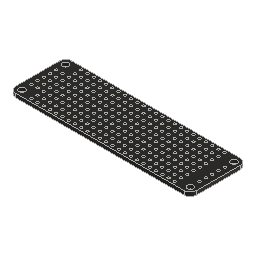
Ingenuity_Micro_Feather_Stacker (Autodesk Fusion 360 design; units mm, degrees)
Autodesk Fusion 360 part; units mm, degrees
sketch "Sketch1" plane through (0, 0, 0) normal (0, 0, 1) x (1, 0, 0) in component "Ingenuity_Micro_Feather_Wing"
  line L0 (36.83, 11.43) -> (-36.83, 11.43)
  line L1 (-36.83, 11.43) -> (-36.83, -11.43)
  line L2 (-36.83, -11.43) -> (36.83, -11.43)
  line L3 (36.83, -11.43) -> (36.83, 11.43)
  line L4 (36.83, 11.43) -> (-36.83, -11.43) construction
  line L5 (-36.83, 11.43) -> (36.83, -11.43) construction
  circle A0 centre (-34.29, 8.89) radius 1.27
  circle A1 centre (-34.29, -8.89) radius 1.27
  line L6 (-36.83, 0) -> (36.83, 0) construction
  line L7 (0, 11.43) -> (0, -11.43) construction
  circle A2 centre (34.29, 8.89) radius 1.27
  circle A3 centre (34.29, -8.89) radius 1.27
  circle A4 centre (-34.29, 0) radius 0.51
  line L8 (-34.29, 8.89) -> (-34.29, -8.89) construction
  circle A5 centre (-34.29, -5.08) radius 0.51
  circle A6 centre (-31.75, -5.08) radius 0.51
  circle A7 centre (-34.29, -2.54) radius 0.51
  circle A8 centre (-31.75, -2.54) radius 0.51
  circle A9 centre (-31.75, 0) radius 0.51
  circle A10 centre (-34.29, 2.54) radius 0.51
  circle A11 centre (-31.75, 2.54) radius 0.51
  circle A12 centre (-34.29, 5.08) radius 0.51
  circle A13 centre (-31.75, 5.08) radius 0.51
  circle A14 centre (-29.21, 0) radius 0.51
  circle A15 centre (-29.21, -10.16) radius 0.51
  circle A16 centre (-26.67, -10.16) radius 0.51
  circle A17 centre (-24.13, -10.16) radius 0.51
  circle A18 centre (-21.59, -10.16) radius 0.51
  circle A19 centre (-19.05, -10.16) radius 0.51
  circle A20 centre (-16.51, -10.16) radius 0.51
  circle A21 centre (-13.97, -10.16) radius 0.51
  circle A22 centre (-11.43, -10.16) radius 0.51
  circle A23 centre (-8.89, -10.16) radius 0.51
  circle A24 centre (-6.35, -10.16) radius 0.51
  circle A25 centre (-3.81, -10.16) radius 0.51
  circle A26 centre (-1.27, -10.16) radius 0.51
  circle A27 centre (1.27, -10.16) radius 0.51
  circle A28 centre (3.81, -10.16) radius 0.51
  circle A29 centre (6.35, -10.16) radius 0.51
  circle A30 centre (8.89, -10.16) radius 0.51
  circle A31 centre (11.43, -10.16) radius 0.51
  circle A32 centre (13.97, -10.16) radius 0.51
  circle A33 centre (16.51, -10.16) radius 0.51
  circle A34 centre (19.05, -10.16) radius 0.51
  circle A35 centre (21.59, -10.16) radius 0.51
  circle A36 centre (24.13, -10.16) radius 0.51
  circle A37 centre (26.67, -10.16) radius 0.51
  circle A38 centre (29.21, -10.16) radius 0.51
  circle A39 centre (-29.21, -7.62) radius 0.51
  circle A40 centre (-26.67, -7.62) radius 0.51
  circle A41 centre (-24.13, -7.62) radius 0.51
  circle A42 centre (-21.59, -7.62) radius 0.51
  circle A43 centre (-19.05, -7.62) radius 0.51
  circle A44 centre (-16.51, -7.62) radius 0.51
  circle A45 centre (-13.97, -7.62) radius 0.51
  circle A46 centre (-11.43, -7.62) radius 0.51
  circle A47 centre (-8.89, -7.62) radius 0.51
  circle A48 centre (-6.35, -7.62) radius 0.51
  circle A49 centre (-3.81, -7.62) radius 0.51
  circle A50 centre (-1.27, -7.62) radius 0.51
  circle A51 centre (1.27, -7.62) radius 0.51
  circle A52 centre (3.81, -7.62) radius 0.51
  circle A53 centre (6.35, -7.62) radius 0.51
  circle A54 centre (8.89, -7.62) radius 0.51
  circle A55 centre (11.43, -7.62) radius 0.51
  circle A56 centre (13.97, -7.62) radius 0.51
  circle A57 centre (16.51, -7.62) radius 0.51
  circle A58 centre (19.05, -7.62) radius 0.51
  circle A59 centre (21.59, -7.62) radius 0.51
  circle A60 centre (24.13, -7.62) radius 0.51
  circle A61 centre (26.67, -7.62) radius 0.51
  circle A62 centre (29.21, -7.62) radius 0.51
  circle A63 centre (-29.21, -5.08) radius 0.51
  circle A64 centre (-26.67, -5.08) radius 0.51
  circle A65 centre (-24.13, -5.08) radius 0.51
  circle A66 centre (-21.59, -5.08) radius 0.51
  circle A67 centre (-19.05, -5.08) radius 0.51
  circle A68 centre (-16.51, -5.08) radius 0.51
  circle A69 centre (-13.97, -5.08) radius 0.51
  circle A70 centre (-11.43, -5.08) radius 0.51
  circle A71 centre (-8.89, -5.08) radius 0.51
  circle A72 centre (-6.35, -5.08) radius 0.51
  circle A73 centre (-3.81, -5.08) radius 0.51
  circle A74 centre (-1.27, -5.08) radius 0.51
  circle A75 centre (1.27, -5.08) radius 0.51
  circle A76 centre (3.81, -5.08) radius 0.51
  circle A77 centre (6.35, -5.08) radius 0.51
  circle A78 centre (8.89, -5.08) radius 0.51
  circle A79 centre (11.43, -5.08) radius 0.51
  circle A80 centre (13.97, -5.08) radius 0.51
  circle A81 centre (16.51, -5.08) radius 0.51
  circle A82 centre (19.05, -5.08) radius 0.51
  circle A83 centre (21.59, -5.08) radius 0.51
  circle A84 centre (24.13, -5.08) radius 0.51
  circle A85 centre (26.67, -5.08) radius 0.51
  circle A86 centre (29.21, -5.08) radius 0.51
  circle A87 centre (-29.21, -2.54) radius 0.51
  circle A88 centre (-26.67, -2.54) radius 0.51
  circle A89 centre (-24.13, -2.54) radius 0.51
  circle A90 centre (-21.59, -2.54) radius 0.51
  circle A91 centre (-19.05, -2.54) radius 0.51
  circle A92 centre (-16.51, -2.54) radius 0.51
  circle A93 centre (-13.97, -2.54) radius 0.51
  circle A94 centre (-11.43, -2.54) radius 0.51
  circle A95 centre (-8.89, -2.54) radius 0.51
  circle A96 centre (-6.35, -2.54) radius 0.51
  circle A97 centre (-3.81, -2.54) radius 0.51
  circle A98 centre (-1.27, -2.54) radius 0.51
  circle A99 centre (1.27, -2.54) radius 0.51
  circle A100 centre (3.81, -2.54) radius 0.51
  circle A101 centre (6.35, -2.54) radius 0.51
  circle A102 centre (8.89, -2.54) radius 0.51
  circle A103 centre (11.43, -2.54) radius 0.51
  circle A104 centre (13.97, -2.54) radius 0.51
  circle A105 centre (16.51, -2.54) radius 0.51
  circle A106 centre (19.05, -2.54) radius 0.51
  circle A107 centre (21.59, -2.54) radius 0.51
  circle A108 centre (24.13, -2.54) radius 0.51
  circle A109 centre (26.67, -2.54) radius 0.51
  circle A110 centre (29.21, -2.54) radius 0.51
  circle A111 centre (-26.67, 0) radius 0.51
  circle A112 centre (-24.13, 0) radius 0.51
  circle A113 centre (-21.59, 0) radius 0.51
  circle A114 centre (-19.05, 0) radius 0.51
  circle A115 centre (-16.51, 0) radius 0.51
  circle A116 centre (-13.97, 0) radius 0.51
  circle A117 centre (-11.43, 0) radius 0.51
  circle A118 centre (-8.89, 0) radius 0.51
  circle A119 centre (-6.35, 0) radius 0.51
  circle A120 centre (-3.81, 0) radius 0.51
  circle A121 centre (-1.27, 0) radius 0.51
  circle A122 centre (1.27, 0) radius 0.51
  circle A123 centre (3.81, 0) radius 0.51
  circle A124 centre (6.35, 0) radius 0.51
  circle A125 centre (8.89, 0) radius 0.51
  circle A126 centre (11.43, 0) radius 0.51
  circle A127 centre (13.97, 0) radius 0.51
  circle A128 centre (16.51, 0) radius 0.51
  circle A129 centre (19.05, 0) radius 0.51
  circle A130 centre (21.59, 0) radius 0.51
  circle A131 centre (24.13, 0) radius 0.51
  circle A132 centre (26.67, 0) radius 0.51
  circle A133 centre (29.21, 0) radius 0.51
  circle A134 centre (-29.21, 2.54) radius 0.51
  circle A135 centre (-26.67, 2.54) radius 0.51
  circle A136 centre (-24.13, 2.54) radius 0.51
  circle A137 centre (-21.59, 2.54) radius 0.51
  circle A138 centre (-19.05, 2.54) radius 0.51
  circle A139 centre (-16.51, 2.54) radius 0.51
  circle A140 centre (-13.97, 2.54) radius 0.51
  circle A141 centre (-11.43, 2.54) radius 0.51
  circle A142 centre (-8.89, 2.54) radius 0.51
  circle A143 centre (-6.35, 2.54) radius 0.51
  circle A144 centre (-3.81, 2.54) radius 0.51
  circle A145 centre (-1.27, 2.54) radius 0.51
  circle A146 centre (1.27, 2.54) radius 0.51
  circle A147 centre (3.81, 2.54) radius 0.51
  circle A148 centre (6.35, 2.54) radius 0.51
  circle A149 centre (8.89, 2.54) radius 0.51
  circle A150 centre (11.43, 2.54) radius 0.51
  circle A151 centre (13.97, 2.54) radius 0.51
  circle A152 centre (16.51, 2.54) radius 0.51
  circle A153 centre (19.05, 2.54) radius 0.51
  circle A154 centre (21.59, 2.54) radius 0.51
  circle A155 centre (24.13, 2.54) radius 0.51
  circle A156 centre (26.67, 2.54) radius 0.51
  circle A157 centre (29.21, 2.54) radius 0.51
  circle A158 centre (-29.21, 5.08) radius 0.51
  circle A159 centre (-26.67, 5.08) radius 0.51
  circle A160 centre (-24.13, 5.08) radius 0.51
  circle A161 centre (-21.59, 5.08) radius 0.51
  circle A162 centre (-19.05, 5.08) radius 0.51
  circle A163 centre (-16.51, 5.08) radius 0.51
  circle A164 centre (-13.97, 5.08) radius 0.51
  circle A165 centre (-11.43, 5.08) radius 0.51
  circle A166 centre (-8.89, 5.08) radius 0.51
  circle A167 centre (-6.35, 5.08) radius 0.51
  circle A168 centre (-3.81, 5.08) radius 0.51
  circle A169 centre (-1.27, 5.08) radius 0.51
  circle A170 centre (1.27, 5.08) radius 0.51
  circle A171 centre (3.81, 5.08) radius 0.51
  circle A172 centre (6.35, 5.08) radius 0.51
  circle A173 centre (8.89, 5.08) radius 0.51
  circle A174 centre (11.43, 5.08) radius 0.51
  circle A175 centre (13.97, 5.08) radius 0.51
  circle A176 centre (16.51, 5.08) radius 0.51
  circle A177 centre (19.05, 5.08) radius 0.51
  circle A178 centre (21.59, 5.08) radius 0.51
  circle A179 centre (24.13, 5.08) radius 0.51
  circle A180 centre (26.67, 5.08) radius 0.51
  circle A181 centre (29.21, 5.08) radius 0.51
  circle A182 centre (-29.21, 7.62) radius 0.51
  circle A183 centre (-26.67, 7.62) radius 0.51
  circle A184 centre (-24.13, 7.62) radius 0.51
  circle A185 centre (-21.59, 7.62) radius 0.51
  circle A186 centre (-19.05, 7.62) radius 0.51
  circle A187 centre (-16.51, 7.62) radius 0.51
  circle A188 centre (-13.97, 7.62) radius 0.51
  circle A189 centre (-11.43, 7.62) radius 0.51
  circle A190 centre (-8.89, 7.62) radius 0.51
  circle A191 centre (-6.35, 7.62) radius 0.51
  circle A192 centre (-3.81, 7.62) radius 0.51
  circle A193 centre (-1.27, 7.62) radius 0.51
  circle A194 centre (1.27, 7.62) radius 0.51
  circle A195 centre (3.81, 7.62) radius 0.51
  circle A196 centre (6.35, 7.62) radius 0.51
  circle A197 centre (8.89, 7.62) radius 0.51
  circle A198 centre (11.43, 7.62) radius 0.51
  circle A199 centre (13.97, 7.62) radius 0.51
  circle A200 centre (16.51, 7.62) radius 0.51
  circle A201 centre (19.05, 7.62) radius 0.51
  circle A202 centre (21.59, 7.62) radius 0.51
  circle A203 centre (24.13, 7.62) radius 0.51
  circle A204 centre (26.67, 7.62) radius 0.51
  circle A205 centre (29.21, 7.62) radius 0.51
  circle A206 centre (-29.21, 10.16) radius 0.51
  circle A207 centre (-26.67, 10.16) radius 0.51
  circle A208 centre (-24.13, 10.16) radius 0.51
  circle A209 centre (-21.59, 10.16) radius 0.51
  circle A210 centre (-19.05, 10.16) radius 0.51
  circle A211 centre (-16.51, 10.16) radius 0.51
  circle A212 centre (-13.97, 10.16) radius 0.51
  circle A213 centre (-11.43, 10.16) radius 0.51
  circle A214 centre (-8.89, 10.16) radius 0.51
  circle A215 centre (-6.35, 10.16) radius 0.51
  circle A216 centre (-3.81, 10.16) radius 0.51
  circle A217 centre (-1.27, 10.16) radius 0.51
  circle A218 centre (1.27, 10.16) radius 0.51
  circle A219 centre (3.81, 10.16) radius 0.51
  circle A220 centre (6.35, 10.16) radius 0.51
  circle A221 centre (8.89, 10.16) radius 0.51
  circle A222 centre (11.43, 10.16) radius 0.51
  circle A223 centre (13.97, 10.16) radius 0.51
  circle A224 centre (16.51, 10.16) radius 0.51
  circle A225 centre (19.05, 10.16) radius 0.51
  circle A226 centre (21.59, 10.16) radius 0.51
  circle A227 centre (24.13, 10.16) radius 0.51
  circle A228 centre (26.67, 10.16) radius 0.51
  circle A229 centre (29.21, 10.16) radius 0.51
  circle A230 centre (34.29, 0) radius 0.51
  circle A231 centre (34.29, -5.08) radius 0.51
  circle A232 centre (34.29, -2.54) radius 0.51
  circle A233 centre (34.29, 2.54) radius 0.51
  circle A234 centre (34.29, 5.08) radius 0.51
  dimension "d1" = 73.66
  dimension "d2" = 22.86
  dimension "d3" = 2.54
  dimension "d4" = 2.54
  dimension "d5" = 2.54
  dimension "d6" = 1.02
  dimension "d10" = 2.54
  dimension "d11" = 2.54
  dimension "d12" = 2.54
  dimension "d15" = 2.54
  dimension "d16" = 2.54
  dimension "d17" = 5.08
  dimension "d20" = 0
  dimension "d21" = 2.54
  constraint horizontal L0
  constraint perpendicular L0 L1
  constraint parallel L0 L2
  constraint parallel L1 L3
  constraint coincident L4 origin
  constraint coincident L5 origin
  constraint equal A0 A1
  constraint midpoint L1 L6.start
  constraint midpoint L3 L6.end
  constraint midpoint L0 L7.start
  constraint midpoint L2 L7.end
  constraint symmetric A0 A1 L6
  constraint equal A0 A2
  constraint symmetric A0 L7 A2
  constraint equal A0 A3
  constraint symmetric A1 L7 A3
  constraint coincident A0.centre L8.start
  constraint coincident A1.centre L8.end
  constraint coincident A4.centre L8
  constraint coincident L6 A4.centre
  constraint coincident L6 A14.centre
  constraint equal A9 A14
  constraint coincident L6 A230.centre
  constraint equal A4 A230
  measures "d1" distance of L1.end L2.end
  measures "d2" distance of L0.end L1.end
  measures "d3" diameter of A0
  measures "d4" distance of L1 A0.centre
  measures "d5" distance of L0 A0.centre
  measures "d6" diameter of A4
  measures "d12" distance of A9.centre A14.centre
  measures "d17" distance of A133.centre A230.centre
extrude "Extrude1" add sketch "Sketch1" along normal blind 1.6 in component "Ingenuity_Micro_Feather_Wing"
fillet "Fillet1" radius 2.54 4 edges at (36.83, -11.43, 0.8) (36.83, 11.43, 0.8) (-36.83, 11.43, 0.8) (-36.83, -11.43, 0.8) in component "Ingenuity_Micro_Feather_Wing"
component "Ingenuity_Micro_Feather_Wing" placed x (1, 0, 0) y (0, 1, 0) z (0, 0, 1) at (0, 0, 0)
